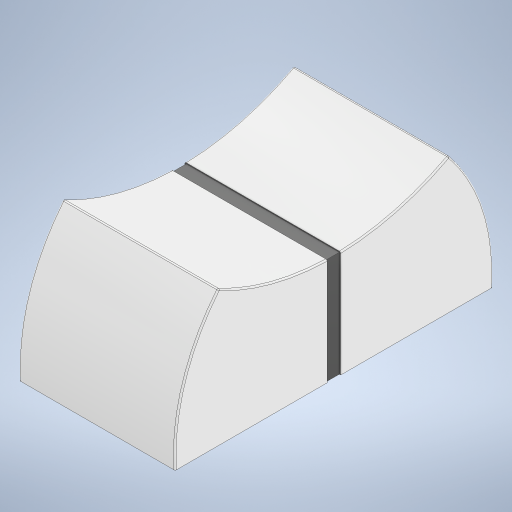
# Autodesk Inventor part: Cup
Saved by Autodesk Inventor 2023 (Build 270158000, 158)
## iProperties
Created: 2024-03-19
Part Number: Cup
Material: Generic
Document SubType Name: Modeling
Designer: noname
Density: 1 g/cm^3
Appearance: PVC - White
Author: noname
Autodesk Inventor part; units mm, degrees
ref_plane "YZ Plane" through (0, 0, 0) normal (1, 0, 0) x (0, 1, 0)
ref_plane "XZ Plane" through (0, 0, 0) normal (0, 1, 0) x (-1, 0, 0)
sketch "Sketch2" plane through (0, 0, 0) normal (1, 0, 0) x (0, 1, 0)
  point P0 (0, 0)
sketch "Sketch3" plane through (0, 0, 0) normal (1, 0, 0) x (0, 1, 0)
  arc A0 (10, 8.5) -> (10, -8.5) centre (25.8666, 0) ccw
  arc A1 (10, 8.5) -> (0, 11.7145) centre (1, -2.3365) ccw
  line L0 (0, 11.7145) -> (0, -11.7145)
  line L1 (0, 0) -> (7.8666, 0)
  line L2 (2.6813, 11.75) -> (0, 11.75) construction
  arc A2 (0, -11.7145) -> (10, -8.5) centre (1, 2.3365) ccw
  line L3 (2.6813, -11.75) -> (0, -11.75) construction
  dimension "d1" = 10
  dimension "d2" = 23.5
  dimension "d3" = 1
  dimension "d4" = 17
  dimension "d5" = 18
  constraints: 8 end point, 7 point on circle, 3 centre point, 3 symmetric about line, 1 coincident, 1 horizontal, 1 midpoint, 1 perpendicular, 1 point on line, 1 tangent, 1 vertical, 1 other
  measures "d1" distance from line of L0 A0.start
  measures "d2" distance of L3.end L2.end
  measures "d3" distance from line of L0 A1.centre
  measures "d4" distance of A0.end A0.start
  measures "d5" radius of A0
extrude "Extrusion1" add sketch "Sketch3" along normal mid plane 11.5
sketch "Sketch4" plane through (-5.75, 0, -11.7145) normal (0, -1, 0) x (1, 0, 0)
  line L0 (4.75, 13.7145) -> (6.75, 13.7145)
  line L1 (6.75, 13.7145) -> (6.75, 9.7145)
  line L2 (6.75, 9.7145) -> (4.75, 9.7145)
  line L3 (4.75, 9.7145) -> (4.75, 13.7145)
  line L4 (4.75, 13.7145) -> (6.75, 9.7145) construction
  line L5 (6.75, 13.7145) -> (4.75, 9.7145) construction
  point P0 (5.75, 11.7145)
  dimension "d8" = 2
  dimension "d9" = 4
  constraints: 12 end point, 2 midpoint, 2 parallel, 1 horizontal, 1 perpendicular
  measures "d8" distance between parallel lines of L3 L1
  measures "d9" distance between parallel lines of L2 L0
extrude "Extrusion2" cut sketch "Sketch4" against normal blind 6
sketch "Sketch5" plane through (5.75, 0, 0) normal (1, 0, 0) x (0, 0, -1)
  line L0 (11.7145, 0) -> (-11.7145, 0) projected
  line L1 (-0.5, 0) -> (0.5, 0)
  line L2 (0.5, 0) -> (0.5, 9.525)
  line L3 (0.5, 9.525) -> (-0.5, 9.525)
  line L4 (-0.5, 9.525) -> (-0.5, 0)
  point P0 (0, 0)
  point P1 (0, 0)
  dimension "d12" = 1
  constraints: 8 end point, 2 midpoint, 2 parallel, 1 horizontal, 1 perpendicular, 1 point on line
  measures "d12" distance between parallel lines of L2 L4
extrude "Extrusion3" cut sketch "Sketch5" against normal blind 0.1
mirror "Mirror1" about plane through (0, 0, 0) normal (1, 0, 0) of "Extrusion3"
ref_plane "Work Plane1" through (5.75, 10, 8.5) normal (0, -1, 0) x (1, 0, 0)
sketch "Sketch6" plane through (5.75, 10, 8.5) normal (0, -1, 0) x (1, 0, 0)
  line L0 (-11.4, -8) -> (-11.4, -9) projected
  line L1 (-11.4, -8) -> (-0.1, -8)
  line L2 (-0.1, -8) -> (-0.1, -9)
  line L3 (-0.1, -9) -> (-11.4, -9)
  line L4 (-11.4, -9) -> (-11.4, -8)
  point P0 (-5.75, -8.5)
  constraints: 8 end point, 2 parallel, 1 coincident, 1 horizontal, 1 perpendicular
extrude "Extrusion4" cut sketch "Sketch6" along normal blind 2.2
fillet "Fillet1" radius 0.1 10 edges at (-5.75, 5.3108, -11.0742) (5.75, 5.3108, -11.0742) (0, 10, -8.5) (5.75, 8.4707, -4.6239) (-5.75, 8.4707, -4.6239) (-5.75, 8.4707, 4.6239) (5.75, 8.4707, 4.6239) (-5.75, 5.3108, 11.0742) (0, 10, 8.5) (5.75, 5.3108, 11.0742)
body "Solid1"
